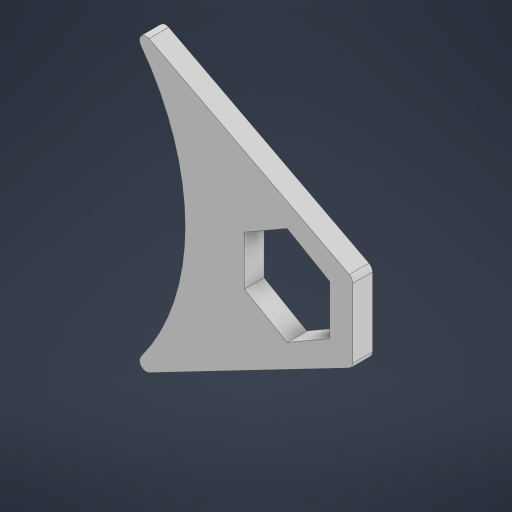
# Autodesk Inventor part: gear-interface
Saved by Autodesk Inventor 2023.2 (Build 272271000, 271)
## iProperties
Created: 2023-03-20
Part Number: gear-interface
Material: Generic
Document SubType Name: Modeling
Designer: Liam
Density: 1 g/cm^3
Appearance: Default
Author: Liam
Autodesk Inventor part; units mm, degrees
ref_plane "YZ Plane" through (0, 0, 0) normal (1, 0, 0) x (0, 1, 0)
ref_plane "XZ Plane" through (0, 0, 0) normal (0, 1, 0) x (-1, 0, 0)
ref_plane "XY Plane" through (0, 0, 0) normal (0, 0, 1) x (1, 0, 0)
sketch "Sketch1" plane through (0, 0, 0) normal (0, 0, 1) x (1, 0, 0)
  circle A0 centre (12.6998, -0.0001) radius 2.0955 projected
  circle A1 centre (12.6998, -0.0001) radius 3.6662
  line L0 (12.6998, -0.0001) -> (25.3998, -0.0001)
  line L1 (12.6998, -0.0001) -> (30.4798, -0.0001)
  line L2 (30.4798, -0.0001) -> (30.4798, 2.6721)
  line L3 (30.4798, -0.0001) -> (30.4798, -2.6723)
  arc A2 (14.0905, -10.422) -> (14.0906, 10.4219) centre (0, 0) ccw
  line L4 (25.3998, 3.8099) -> (28.6994, 1.9049)
  line L5 (28.6994, -1.9051) -> (28.6994, 1.9049)
  line L6 (28.6994, -1.9051) -> (25.3998, -3.8101)
  line L7 (22.1003, -1.9051) -> (25.3998, -3.8101)
  line L8 (22.1003, -1.9051) -> (22.1003, 1.9049)
  line L9 (25.3998, 3.8099) -> (22.1003, 1.9049)
  line L10 (14.7335, 11.1746) -> (30.2063, 3.1227)
  line L11 (14.7334, -11.1747) -> (30.2063, -3.1229)
  arc A3 (14.7335, 11.1746) -> (14.0906, 10.4219) centre (14.499, 10.724) ccw
  arc A4 (14.0905, -10.422) -> (14.7334, -11.1747) centre (14.4989, -10.7241) ccw
  arc A5 (30.2063, -3.1229) -> (30.4798, -2.6723) centre (29.9718, -2.6723) ccw
  arc A6 (30.4798, 2.6721) -> (30.2063, 3.1227) centre (29.9718, 2.6721) ccw
  point P0 (12.6998, 3.6661)
  point P1 (16.4691, 5.9941)
  point P2 (16.469, -5.9943)
  point P3 (30.4798, 5.0799)
  point P4 (30.4798, -5.0801)
  point P5 (12.3928, 12.3927)
  point P6 (12.3927, -12.3928)
  dimension "d3" = 12.7
  dimension "d10" = 17.78
  dimension "d11" = 5.08
  dimension "d12" = 5.08
  dimension "d19" = 3.81
  dimension "d24" = 0.508
  constraints: 24 end point, 12 point on circle, 8 tangent, 5 centre point, 5 point on line, 5 vertical, 3 equal radius, 3 parallel, 1 coincident, 1 horizontal, 1 vertical alignment, 7 other
  measures "d3" distance of L0.start L0.end
  measures "d10" distance of L0.start L1.end
  measures "d11" distance of L1.end point (30.48, 5.08)
  measures "d12" distance of L1.end point (30.48, -5.08)
  measures "d19" distance of L0.end L4.start
  measures "d24" radius of A3
extrude "Extrusion2" add sketch "Sketch1" along normal blind 1.524 contours A2 A3 L10 A6 L2 L1 L5 L4 L9 L8 L0 | L0 L8 L7 L6 L5 L1 L3 A5 L11 A4 A2
body "Solid2"
